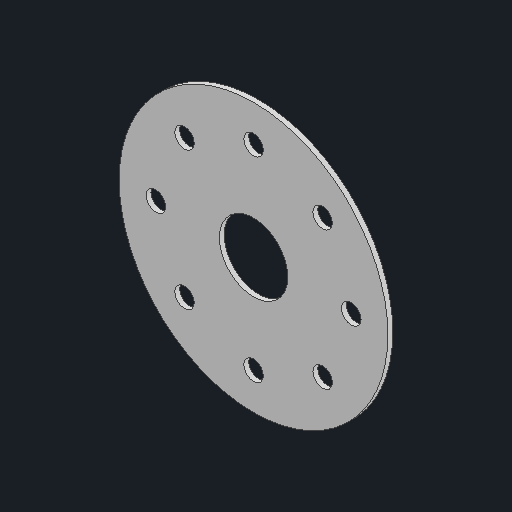
# Autodesk Inventor part: DMF flange small gear
Saved by Autodesk Inventor 2026.2 (Build 302298000, 298)
## iProperties
Created: 2024-04-30
Part Number: DMF flange small gear
Material: Generic
Document SubType Name: Sheet Metal
Designer: pokla
Stock Number: Барабан_Сектор_Усилителя
Density: 1 g/cm^3
Sheet Metal Rule: Default
Sheet Metal Width: 0,000 mm
Sheet Metal Length: 0,000 mm
Sheet Metal Area: 0,000 mm^2
Appearance: Default
Author: pokla
Autodesk Inventor part; units mm, degrees
ref_plane "YZ Plane" through (0, 0, 0) normal (1, 0, 0) x (0, 1, 0)
ref_plane "XZ Plane" through (0, 0, 0) normal (0, 1, 0) x (-1, 0, 0)
ref_plane "XY Plane" through (0, 0, 0) normal (0, 0, 1) x (1, 0, 0)
sketch "Sketch1" plane through (0, 0, 0) normal (0, 0, 1) x (1, 0, 0)
  circle A0 centre (0, 0) radius 55
  circle A1 centre (0, 0) radius 14
  circle A2 centre (0, 0) radius 40 construction
  circle A3 centre (40, 0) radius 4
  circle A4 centre (28.2843, 28.2843) radius 4
  circle A5 centre (0, 40) radius 4
  circle A6 centre (-28.2843, 28.2843) radius 4
  circle A7 centre (-40, 0) radius 4
  circle A8 centre (-28.2843, -28.2843) radius 4
  circle A9 centre (0, -40) radius 4
  circle A10 centre (28.2843, -28.2843) radius 4
  dimension "d39" = 80
  dimension "d31" = 28
  dimension "d32" = 110
  dimension "d40" = 8
  dimension "d43" = 360
  measures "d31" diameter of A1
  measures "d32" diameter of A0
  measures "d40" diameter of A3
extrude "Plate1" add sketch "Sketch1" against normal blind 2
equation "\"d15\" = Thickness"
equation "\"BendRadius\" = Thickness"
equation "\"BendReliefWidth\" = Thickness"
equation "\"BendReliefDepth\" = 0.5 * Thickness"
equation "\"CornerReliefSize\" = 4 * Thickness"
equation "\"MinimumRemnant\" = 2 * Thickness"
equation "\"TransitionRadius\" = BendRadius"
equation "\"JacobiRadiusSize\" = BendRadius"
equation "\"GapSize\" = Thickness"
equation "\"Thickness\" = 2"
body "Solid1"
